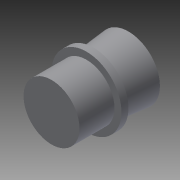
# Autodesk Inventor part: backtop
Saved by Autodesk Inventor 2015 (Build 190159000, 159)
## iProperties
Created: 2014-11-30
Part Number: backtop
Material: 常规
Document SubType Name: Modeling
Designer: zenkr
Density: 1 g/cm^3
Appearance: 默认
Author: zenkr
Autodesk Inventor part; units mm, degrees
ref_plane "YZ Plane" through (0, 0, 0) normal (1, 0, 0) x (0, 1, 0)
ref_plane "XZ Plane" through (0, 0, 0) normal (0, 1, 0) x (-1, 0, 0)
sketch "草图1" plane through (0, 0, 0) normal (0, 1, 0) x (-1, 0, 0)
  circle A0 centre (0, 0) radius 5
  dimension "d0" = 10
  constraints: 1 centre point, 1 coincident
  measures "d0" diameter of A0
extrude "拉伸1" add sketch "草图1" along normal blind 1
sketch "草图2" plane through (0, 1, 0) normal (0, 1, 0) x (1, 0, 0)
  circle A0 centre (0, 0) radius 4
  dimension "d3" = 8
  constraints: 1 centre point, 1 coincident
  measures "d3" diameter of A0
ref_plane "工作平面1" through (0, 6, 0) normal (0, 1, 0) x (1, 0, 0)
sketch "草图3" plane through (0, 6, 0) normal (0, 1, 0) x (1, 0, 0)
  circle A0 centre (0, 0) radius 4.5
  dimension "d5" = 9
  constraints: 1 centre point, 1 coincident
  measures "d5" diameter of A0
loft "放样1" add profiles "草图2", "草图3"
sketch "草图4" plane through (0, 0, 0) normal (0, -1, 0) x (1, 0, 0)
  circle A0 centre (0, 0) radius 4
  dimension "d11" = 8
  constraints: 1 centre point, 1 coincident
  measures "d11" diameter of A0
extrude "拉伸2" add sketch "草图4" along normal blind 5
